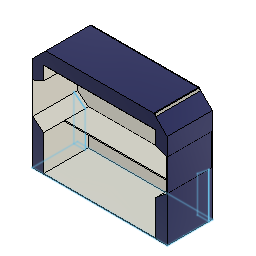
f1-pit-display (Autodesk Fusion 360 design; units mm, degrees)
Autodesk Fusion 360 part; units mm, degrees
sketch "Sketch1" plane through (0, 0, 0) normal (0, 0, 1) x (1, 0, 0)
  line L0 (-100, 80) -> (2900, 80)
  line L1 (2900, 80) -> (2900, -920)
  line L2 (2900, -920) -> (-100, -920)
  line L3 (-100, -920) -> (-100, 80)
  dimension "d1" = 3000
  dimension "d2" = 1000
  constraint horizontal L0
  constraint vertical L1
  constraint horizontal L2
  constraint vertical L3
  measures "d1" distance of L0.start L0.end
  measures "d2" distance of L0.start L2.end
extrude "Extrude1" add sketch "Sketch1" along normal blind 10 makes body 1
sketch "Sketch2" plane through (0, 0, 0) normal (1, 0, 0) x (0, 1, 0)
sketch "Sketch3" plane through (0, 0, 0) normal (0, 1, 0) x (1, 0, 0)
  line L0 (-100, 0) -> (-100, -1000)
  line L1 (-100, -1000) -> (150, -800)
  line L2 (150, -800) -> (150, 0)
  line L3 (2900, 0) -> (2900, -1000)
  line L4 (2650, -800) -> (2650, 0)
  line L5 (2900, -1000) -> (2650, -800)
  line L6 (-100, 0) -> (150, 0)
  line L7 (2650, 0) -> (2900, 0)
  dimension "d5" = 1000
  constraint vertical L0
  constraint parallel L0 L2
  constraint perpendicular L2 L6
  constraint perpendicular L3 L7
  measures "d5" distance of L0.start L0.end
extrude "Extrude2" add sketch "Sketch3" along normal blind 80 contours L3 L4 L5 L7 bodies 1
extrude "Extrude3" add sketch "Sketch3" along normal blind 80 contours L0 L1 L2 L6 bodies 1
extrude "Extrude4" add sketch "Sketch3" against normal blind 925 contours L3 L4 L5 L7 bodies 1
extrude "Extrude5" add sketch "Sketch3" against normal blind 925 contours L0 L1 L2 L6 bodies 1
ref_plane "WorkPlane1" through (0, 0, 0) normal (1, 0, 0) x (0, 1, 0)
ref_plane "WorkPlane2" through (-100, 0, 0) normal (1, 0, 0) x (0, 1, 0)
ref_plane "WorkPlane3" through (2900, 0, 0) normal (1, 0, 0) x (0, 1, 0)
sketch "Sketch4" plane through (2900, 0, 0) normal (1, 0, 0) x (0, 1, 0)
  line L0 (-925, 0) -> (75, 0)
  line L1 (75, 0) -> (75, 2400)
  line L2 (75, 2400) -> (-925, 2400)
  line L3 (-925, 2400) -> (-925, 0)
  dimension "d17" = 1000
  dimension "d18" = 2400
  constraint horizontal L0
  constraint vertical L1
  constraint horizontal L2
  constraint vertical L3
  measures "d17" distance of L0.start L0.end
  measures "d18" distance of L0.start L2.end
sketch "Sketch5" plane through (-100, 0, 0) normal (1, 0, 0) x (0, 1, 0)
  line L0 (80, 0) -> (-920, 0)
  line L1 (-920, 0) -> (-920, 2400)
  line L2 (-920, 2400) -> (80, 2400)
  line L3 (80, 2400) -> (80, 0)
  dimension "d19" = 1000
  dimension "d20" = 2400
  constraint horizontal L0
  constraint vertical L1
  constraint horizontal L2
  constraint vertical L3
  measures "d19" distance of L0.start L0.end
  measures "d20" distance of L0.start L2.end
extrude "Extrude6" add sketch "Sketch5" along normal blind 10 bodies 1
extrude "Extrude7" add sketch "Sketch4" against normal blind 10 bodies 1
sketch "Sketch6" plane through (0, -925, 0) normal (0, -1, 0) x (1, 0, 0)
  line L0 (2890, 992) -> (2650, 800)
  line L1 (2650, 800) -> (2650, 0)
  line L2 (2650, 0) -> (2900, 0)
  line L3 (2900, 0) -> (2900, 2400)
  line L4 (2900, 2400) -> (2890, 2400)
  line L5 (2890, 2400) -> (2890, 992)
  line L6 (2890, 2400) -> (2644.5768, 2400)
  line L7 (2644.5768, 2400) -> (2644.5768, 1800)
  line L8 (2644.5768, 1800) -> (2890, 1696)
  line L9 (2890, 1696) -> (2890, 2400)
  line L10 (155.4232, 2400) -> (155.4232, 1800)
  line L11 (155.4232, 1800) -> (-90, 1696)
  line L12 (-90, 2400) -> (155.4232, 2400)
  line L13 (-90, 1696) -> (-90, 2400)
  constraint coincident L4.end L5.start
  constraint perpendicular L5 L6
  constraint perpendicular L6 L7
  constraint midpoint L5 L8.end
extrude "Extrude8" add sketch "Sketch6" against normal blind 1000 contours L5 L6 L7 L8 L9 | L10 L11 L12 L13 bodies 1
sketch "Sketch7" plane through (0, -925, 0) normal (0, -1, 0) x (1, 0, 0)
  line L0 (2890, 992) -> (2650, 800)
  line L1 (2650, 800) -> (2650, 0)
  line L2 (2650, 0) -> (2900, 0)
  line L3 (2900, 0) -> (2900, 2400)
  line L4 (2900, 2400) -> (2644.5768, 2400)
  line L5 (2644.5768, 2400) -> (2644.5768, 1800)
  line L6 (2644.5768, 1800) -> (2890, 1696)
  line L7 (2890, 1696) -> (2890, 992)
  line L8 (-100, 2400) -> (2900, 2400)
  line L9 (2900, 2400) -> (2900, 2100)
  line L10 (2900, 2100) -> (-100, 2100)
  line L11 (-100, 2100) -> (-100, 2400)
  dimension "d27" = 3000
  dimension "d28" = 300
  constraint horizontal L8
  constraint vertical L9
  constraint horizontal L10
  constraint vertical L11
  measures "d27" distance of L8.start L3.end
  measures "d28" distance of L8.start L10.end
extrude "Extrude9" add sketch "Sketch7" against normal blind 10 contours L5 L8 L10 L11 | L3 L4 L5 L8 L9 L10 bodies 1
sketch "Sketch8" plane through (0, 80, 0) normal (0, 1, 0) x (-1, 0, 0)
  line L0 (90, 992) -> (-150, 800)
  line L1 (-150, 800) -> (-150, 10)
  line L2 (-150, 10) -> (-2650, 10)
  line L3 (-2650, 10) -> (-2650, 800)
  line L4 (-2650, 800) -> (-2900, 1000)
  line L5 (-2900, 1000) -> (-2900, 0)
  line L6 (-2900, 0) -> (100, 0)
  line L7 (100, 0) -> (100, 2400)
  line L8 (100, 2400) -> (90, 2400)
  line L9 (90, 2400) -> (90, 992)
  line L10 (-2900, 0) -> (90, 0)
  line L11 (90, 0) -> (90, 2400)
  line L12 (90, 2400) -> (-2900, 2400)
  line L13 (-2900, 2400) -> (-2900, 0)
  constraint horizontal L10
  constraint vertical L11
  constraint horizontal L12
  constraint vertical L13
  constraint coincident L8.end L9.start
  constraint coincident L5.end L6.start
extrude "Extrude10" add sketch "Sketch8" against normal blind 10 contours L0 L1 L2 L3 L4 L9 L11 L12 L13 bodies 1
sketch "Sketch9" plane through (0, 0, 2400) normal (0, 0, 1) x (-1, 0, 0)
  line L0 (-2644.5768, -70) -> (-2644.5768, 915)
  line L1 (-2644.5768, 915) -> (-155.4232, 915)
  line L2 (-155.4232, 915) -> (-155.4232, -70)
  line L3 (-155.4232, -70) -> (-2644.5768, -70)
  line L4 (-2900, 925) -> (-2900, -80)
  line L5 (-2900, -80) -> (100, -80)
  line L6 (100, -80) -> (100, 925)
  line L7 (100, 925) -> (-2900, 925)
  line L8 (100, -80) -> (-2900, -80)
  line L9 (-2900, -80) -> (-2900, 925)
  line L10 (-2900, 925) -> (100, 925)
  line L11 (100, 925) -> (100, -80)
  constraint horizontal L8
  constraint vertical L9
  constraint horizontal L10
  constraint vertical L11
  constraint coincident L4.start L7.end
  constraint coincident L5.end L6.start
extrude "Extrude11" add sketch "Sketch9" against normal blind 10 contours L0 L1 L2 L3 | L4 L5 L6 L7 L8 L9 L10 L11 bodies 1
sketch "Sketch10" plane through (0, -925, 0) normal (0, -1, 0) x (1, 0, 0)
  line L0 (-100, 2400) -> (-100, 2100)
  line L1 (-100, 2100) -> (-90, 2100)
  line L2 (-90, 2100) -> (-90, 1696)
  line L3 (-90, 1696) -> (155.4232, 1800)
  line L4 (155.4232, 1800) -> (155.4232, 2100)
  line L5 (155.4232, 2100) -> (2644.5768, 2100)
  line L6 (2644.5768, 2100) -> (2644.5768, 1800)
  line L7 (2644.5768, 1800) -> (2890, 1696)
  line L8 (2890, 1696) -> (2890, 992)
  line L9 (2890, 992) -> (2650, 800)
  line L10 (2650, 800) -> (2650, 0)
  line L11 (2650, 0) -> (2900, 0)
  line L12 (2900, 0) -> (2900, 2400)
  line L13 (2900, 2400) -> (-100, 2400)
  line L14 (-100, 2100) -> (200, 2400)
  line L15 (-100, 2400) -> (-100, 2100)
  line L16 (-100, 2400) -> (200, 2400)
  line L17 (2900, 2100) -> (2600, 2400)
  line L18 (2900, 2400) -> (2900, 2100)
  line L19 (2900, 2400) -> (2600, 2400)
  line L20 (-90, 1978.4213) -> (200, 2400)
  line L21 (200, 2400) -> (-100, 2400)
  line L22 (-100, 2400) -> (-100, 1978.4213)
  line L23 (-100, 1978.4213) -> (200, 2400)
  line L24 (200, 2400) -> (-100, 2400)
  constraint coincident L0.end L1.start
  constraint coincident L13 L14.end
  constraint coincident L0.start L13.end
  constraint coincident L2 L20.start
  constraint perpendicular L21 L22
sketch "Sketch11" plane through (0, 0, 0) normal (0, 1, 0) x (1, 0, 0)
  line L0 (-100, -2100) -> (200, -2400)
  line L1 (200, -2400) -> (-100, -2400)
  line L2 (-100, -2400) -> (-100, -2100)
  line L3 (2900, -2400) -> (2600, -2400)
  line L4 (2600, -2400) -> (2900, -2100)
  line L5 (2900, -2100) -> (2900, -2400)
  constraint horizontal L1
  constraint perpendicular L1 L2
  constraint perpendicular L2 L3
  constraint perpendicular L0 L4
  constraint perpendicular L3 L5
extrude "Extrude12" cut sketch "Sketch11" along normal blind 1500 and the other way blind 2000 bodies 1
ref_plane "WorkPlane4" through (0, 0, 800) normal (0, 0, 1) x (1, 0, 0)
sketch "Sketch12" plane through (0, 0, 800) normal (0, 0, 1) x (1, 0, 0)
  line L0 (199.3612, 79.0385) -> (2600, 79.0385)
  line L1 (2600, 79.0385) -> (2600, -450)
  line L2 (2600, -450) -> (199.3612, -450)
  line L3 (199.3612, -450) -> (199.3612, 79.0385)
  constraint horizontal L0
  constraint vertical L1
  constraint horizontal L2
  constraint vertical L3
extrude "Extrude13" add sketch "Sketch12" against normal blind 25 separate body makes body 2
scale "Scale1" factors (1.1, 1, 1) about (199.3612, 79.0385, 800) bodies 2
move_body "Move1" bodies 2 to x (1, 0, 0) y (0, 1, 0) z (0, 0, 1) at (-100, 0, 0)
